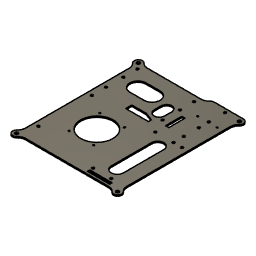
MoBo (Autodesk Fusion 360 archive; units mm, degrees)
design "MoBo"
Autodesk Fusion 360 part; units mm, degrees
sketch "Sketch1" plane through (0, 0, 0) normal (0, 1, 0) x (1, 0, 0)
  arc A0 (25.8589, 127) -> (18.199, 123.4286) centre (25.8589, 117) ccw
  circle A1 centre (62, 16) radius 3
  arc A2 (4.4113, 117) -> (18.199, 123.4286) centre (4.4113, 135) ccw
  line L0 (-64.5, 44) -> (-99.5, 44)
  line L1 (-151.5, 95.5524) -> (-151.5, -162.5524)
  line L2 (98.5, -162.5524) -> (98.5, 95.5524)
  line L3 (-31.5, 36) -> (-31.5, 54)
  circle A3 centre (-151.5, -184) radius 4
  arc A4 (-130.0524, -184) -> (-143.8401, -190.4286) centre (-130.0524, -202) ccw
  line L4 (-13.5, 4) -> (-69.5, 4)
  line L5 (-69.5, 19) -> (-13.5, 19)
  line L6 (-69.5, 4) -> (-69.5, 19)
  circle A5 centre (62.5, -10) radius 3
  line L7 (-130.0524, -184) -> (77.0524, -184)
  circle A6 centre (83.5, -10) radius 3
  line L8 (4.4113, 117) -> (-130.0524, 117)
  circle A7 centre (0.5, 103) radius 3
  circle A8 centre (62, 53) radius 3
  arc A9 (-157.9286, -176.3401) -> (-143.8401, -190.4286) centre (-151.5, -184) ccw
  arc A10 (-151.5, 95.5524) -> (-157.9286, 109.3401) centre (-169.5, 95.5524) ccw
  arc A11 (104.9286, 109.3401) -> (98.5, 127) centre (98.5, 117) ccw
  circle A12 centre (-139.5, 103) radius 3
  arc A13 (104.9286, 109.3401) -> (98.5, 95.5524) centre (116.5, 95.5524) ccw
  arc A14 (-5.5, 54) -> (-31.5, 54) centre (-18.5, 54) ccw
  circle A15 centre (0.5, 25) radius 3
  arc A16 (-31.5, 36) -> (-5.5, 36) centre (-18.5, 36) ccw
  circle A17 centre (98.5, 117) radius 4
  circle A18 centre (17.5, -10) radius 3
  circle A19 centre (-151.5, 117) radius 4
  circle A20 centre (-139.5, 25) radius 3
  circle A21 centre (62.5, -164) radius 3
  arc A22 (-157.9286, -176.3401) -> (-151.5, -162.5524) centre (-169.5, -162.5524) ccw
  arc A23 (98.5, -162.5524) -> (104.9286, -176.3401) centre (116.5, -162.5524) ccw
  arc A24 (65.5, -37) -> (35.5, -37) centre (50.5, -37) ccw
  line L9 (65.5, -37) -> (65.5, -137)
  line L10 (35.5, -137) -> (35.5, -37)
  arc A25 (35.5, -137) -> (65.5, -137) centre (50.5, -137) ccw
  circle A26 centre (98.5, -184) radius 4
  circle A27 centre (-30.5, -114) radius 2
  circle A28 centre (17.5, -164) radius 3
  circle A29 centre (-91.5, -114) radius 2
  arc A30 (90.8401, -190.4286) -> (77.0524, -184) centre (77.0524, -202) ccw
  arc A31 (90.8401, -190.4286) -> (104.9286, -176.3401) centre (98.5, -184) ccw
  circle A32 centre (-61, -76) radius 40
  circle A33 centre (-30.5, -38) radius 2
  circle A34 centre (-91.5, -38) radius 2
  circle A35 centre (-139.5, -142) radius 3
  circle A36 centre (62, 118) radius 3
  arc A37 (-64.5, 44) -> (-64.5, 84) centre (-64.5, 64) ccw
  line L11 (16.5, 56.5) -> (24.5, 56.5)
  circle A38 centre (-139.5, -10) radius 3
  line L12 (16.5, 16.5) -> (16.5, 56.5)
  line L13 (98.5, 127) -> (25.8589, 127)
  line L14 (-99.5, 84) -> (-64.5, 84)
  line L15 (-13.5, 19) -> (-13.5, 4)
  arc A39 (-143.8401, 123.4286) -> (-157.9286, 109.3401) centre (-151.5, 117) ccw
  arc A40 (-143.8401, 123.4286) -> (-130.0524, 117) centre (-130.0524, 135) ccw
  arc A41 (-99.5, 84) -> (-99.5, 44) centre (-99.5, 64) ccw
  line L16 (24.5, 56.5) -> (24.5, 16.5)
  line L17 (-5.5, 54) -> (-5.5, 36)
  line L18 (24.5, 16.5) -> (16.5, 16.5)
  line L19 (-34.0405, 19) -> (-13.5, 11.5)
  line L20 (62.5, -164) -> (72.5, -164) construction
  line L21 (72.5, -164) -> (72.5, -172) construction
  line L22 (72.5, -172) -> (62.5, -172) construction
  line L23 (62.5, -172) -> (62.5, -164) construction
  line L24 (17.5, -164) -> (17.5, -172) construction
  line L25 (17.5, -172) -> (72.5, -172)
  line L26 (72.5, -172) -> (72.5, -178.01)
  line L27 (72.5, -178.01) -> (17.5, -178.01)
  line L28 (17.5, -178.01) -> (17.5, -172)
  circle A42 centre (36, 76.5) radius 2
  circle A43 centre (84, 76.5) radius 2
  circle A44 centre (-139.5, 68) radius 3
  circle A45 centre (0.5, 68) radius 3
  circle A46 centre (62, 78) radius 3
  point P0 (-61, -76)
  dimension "d5" = 10
  dimension "d6" = 8
  dimension "d7" = 8
  dimension "d8" = 6.01
  dimension "d9" = 4
  dimension "d10" = 48
  constraint coincident L5 L19.start
  constraint midpoint L15 L19.end
  constraint horizontal L20
  constraint vertical L21
  constraint horizontal L22
  constraint vertical L23
  constraint coincident A21.centre L20.start
  constraint vertical L24
  constraint coincident A28.centre L24.start
  constraint horizontal L25
  constraint vertical L26
  constraint horizontal L27
  constraint vertical L28
  constraint coincident L21.end L22.start
  measures "d5" distance of A21.centre L20.end
  measures "d6" distance of A21.centre L22.end
  measures "d7" distance of A28.centre L24.end
  measures "d8" distance of L24.end L27.end
  measures "d9" diameter of A42
  measures "d10" distance of A43.centre A42.centre
extrude "Extrude1" add sketch "Sketch1" along normal blind 3 contours A0 A2 L1 L2 A4 L7 L8 A9 A10 A11 A13 A22 A23 A30 A31 L13 A39 A40 | L5 L15 L19
equation "d7 = d6"
